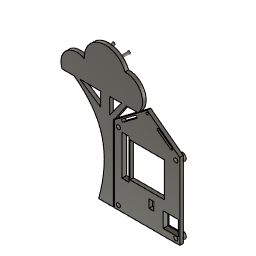
FaceCover v11 (Autodesk Fusion 360 design; units mm, degrees)
Autodesk Fusion 360 part; units mm, degrees
note: some values were not read from the file. Set by a fixed rule: which sketch regions a step uses.
sketch "House" plane through (0, 0, 0) normal (0, 1, 0) x (1, 0, 0)
  line L0 (27.95, 32.5) -> (-27.95, 32.5)
  line L1 (-27.95, 32.5) -> (-27.95, -32.5)
  line L2 (-27.95, -32.5) -> (27.95, -32.5)
  line L3 (27.95, -32.5) -> (27.95, 32.5)
  line L4 (27.95, 32.5) -> (-27.95, -32.5) construction
  line L5 (-27.95, 32.5) -> (27.95, -32.5) construction
  line L6 (14.8, 5.3) -> (-14.7, 5.3)
  line L7 (-14.7, 5.3) -> (-14.7, -24.2)
  line L8 (-14.7, -24.2) -> (14.8, -24.2)
  line L9 (14.8, -24.2) -> (14.8, 5.3)
  line L10 (14.8, 5.3) -> (-14.7, -24.2) construction
  line L11 (-14.7, 5.3) -> (14.8, -24.2) construction
  circle A0 centre (-24.45, 29) radius 1.75
  circle A1 centre (-24.45, -28.7) radius 1.75
  line L12 (-24.45, 29) -> (-24.45, -28.7) construction
  circle A2 centre (24.55, 29) radius 1.75
  line L13 (-24.45, 29) -> (24.55, 29) construction
  circle A3 centre (24.55, -28.7) radius 1.75
  line L14 (-24.45, -28.7) -> (24.55, -28.7) construction
  line L15 (24.55, -28.7) -> (24.55, 29) construction
  line L16 (-15.45, -24.5) -> (-19.45, -24.5)
  line L17 (-19.45, -24.5) -> (-19.45, 5.5)
  line L18 (-19.45, 5.5) -> (-15.45, 5.5)
  line L19 (-15.45, 5.5) -> (-15.45, -24.5)
  line L20 (15.7, 16) -> (24.7, 16)
  line L21 (24.7, 16) -> (24.7, 25)
  line L22 (24.7, 25) -> (15.7, 25)
  line L23 (15.7, 25) -> (15.7, 16)
  line L24 (1.65, 11.25) -> (5.65, 11.25)
  line L25 (5.65, 11.25) -> (5.65, 18.25)
  line L26 (5.65, 18.25) -> (1.65, 18.25)
  line L27 (1.65, 18.25) -> (1.65, 11.25)
  point P0 (0.05, -9.45)
  dimension "d1" = 55.9
  dimension "d2" = 65
  dimension "d3" = 29.5
  dimension "d4" = 29.5
  dimension "d5" = 27.2
  dimension "d7" = 3.5
  dimension "d8" = 3.5
  dimension "d10" = 57.7
  dimension "d12" = 49
  dimension "d13" = 3.5
  dimension "d14" = 4
  dimension "d15" = 30
  dimension "d16" = 8.5
  dimension "d17" = 27
  dimension "d18" = 9
  dimension "d19" = 9
  dimension "d20" = 7.5
  dimension "d21" = 3.25
  dimension "d22" = 4
  dimension "d23" = 7
  dimension "d24" = 14.25
  dimension "d25" = 22.3
  dimension "d92" = 28
  constraint horizontal L0
  constraint perpendicular L0 L1
  constraint parallel L0 L2
  constraint parallel L1 L3
  constraint coincident L4 origin
  constraint coincident L5 origin
  constraint horizontal L6
  constraint perpendicular L6 L7
  constraint parallel L6 L8
  constraint parallel L7 L9
  constraint coincident L10 P0
  constraint coincident L11 P0
  constraint coincident A0.centre L12.start
  constraint coincident A1.centre L12.end
  constraint vertical L12
  constraint coincident A2.centre L13.end
  constraint parallel L0 L13
  constraint coincident A3.centre L14.end
  constraint vertical L15
  constraint horizontal L16
  constraint vertical L17
  constraint horizontal L18
  constraint vertical L19
  constraint horizontal L20
  constraint vertical L21
  constraint horizontal L22
  constraint vertical L23
  constraint horizontal L24
  constraint vertical L25
  constraint horizontal L26
  constraint vertical L27
  constraint equal A1 A3
  constraint equal A0 A1
  constraint equal A0 A2
  measures "d1" distance of L1.end L2.end
  measures "d2" distance of L0.end L1.end
  measures "d3" distance of L7.end L8.end
  measures "d4" distance of L6.start L8.end
  measures "d5" distance of L0 L6
  measures "d7" distance of L0 A0.centre
  measures "d8" distance of L1 A0.centre
  measures "d10" distance of A0.centre A1.centre
  measures "d12" distance of A0.centre A2.centre
  measures "d13" diameter of A3
  measures "d14" distance of L16.start L16.end
  measures "d15" distance of L16.start L18.end
  measures "d16" distance of L1 L17
  measures "d17" distance of L0 L18
  measures "d18" distance of L20.start L20.end
  measures "d19" distance of L20.start L22.end
  measures "d20" distance of L0 L22
  measures "d21" distance of L3 L21
  measures "d22" distance of L24.start L24.end
  measures "d23" distance of L24.start L26.end
  measures "d24" distance of L0 L26
  measures "d25" distance of L3 L25
  measures "d92" distance of L1 P0
extrude "Extrude1" add sketch "House" along normal blind 3 makes body 1
sketch "Roof" plane through (0, 0, 0) normal (0, -1, 0) x (1, 0, 0)
  circle A0 centre (24.55, -29) radius 1.75
  line L0 (14.8, 24.2) -> (14.8, -5.3)
  line L1 (14.8, -5.3) -> (-14.7, -5.3)
  line L2 (-14.7, -5.3) -> (-14.7, 24.2)
  line L3 (-14.7, 24.2) -> (14.8, 24.2)
  circle A1 centre (-24.45, 28.7) radius 1.75
  circle A2 centre (-24.45, -29) radius 1.75
  circle A3 centre (24.55, 28.7) radius 1.75
  line L4 (-15.45, -5.5) -> (-19.45, -5.5)
  line L5 (-19.45, -5.5) -> (-19.45, 24.5)
  line L6 (-19.45, 24.5) -> (-15.45, 24.5)
  line L7 (-15.45, 24.5) -> (-15.45, -5.5)
  line L8 (15.7, -25) -> (15.7, -16)
  line L9 (15.7, -16) -> (24.7, -16)
  line L10 (24.7, -16) -> (24.7, -25)
  line L11 (24.7, -25) -> (15.7, -25)
  line L12 (1.65, -18.25) -> (1.65, -11.25)
  line L13 (1.65, -11.25) -> (5.65, -11.25)
  line L14 (5.65, -11.25) -> (5.65, -18.25)
  line L15 (5.65, -18.25) -> (1.65, -18.25)
  line L16 (27.95, -32.5) -> (27.95, 32.5)
  line L17 (27.95, 32.5) -> (-27.95, 32.5)
  line L18 (-27.95, 32.5) -> (-27.95, -32.5)
  line L19 (-27.95, -32.5) -> (27.95, -32.5)
  line L20 (-27.95, 32.5) -> (0, 53.5)
  line L21 (0, 53.5) -> (27.95, 32.5)
  line L22 (0, 0) -> (0, 2.2581) construction
  line L23 (0, 2.2581) -> (0, 69.3742) construction
  dimension "d28" = 21
  constraint coincident L17.end L18.start
  constraint coincident L16.end L17.start
  constraint coincident L22.start origin
  constraint perpendicular L1 L22
  constraint parallel L0 L23
  constraint coincident L20.end L23
  measures "d28" distance of L17 L20.end
extrude "Extrude2" add sketch "Roof" against normal blind 3 contours L17 L20 L21 bodies 1
sketch "Chimney" plane through (0, 0, 0) normal (0, -1, 0) x (1, 0, 0)
  circle A0 centre (24.55, -29) radius 1.75
  line L0 (14.8, 24.2) -> (14.8, -5.3)
  line L1 (14.8, -5.3) -> (-14.7, -5.3)
  line L2 (-14.7, -5.3) -> (-14.7, 24.2)
  line L3 (-14.7, 24.2) -> (14.8, 24.2)
  circle A1 centre (-24.45, 28.7) radius 1.75
  circle A2 centre (-24.45, -29) radius 1.75
  circle A3 centre (24.55, 28.7) radius 1.75
  line L4 (-15.45, -5.5) -> (-19.45, -5.5)
  line L5 (-19.45, -5.5) -> (-19.45, 24.5)
  line L6 (-19.45, 24.5) -> (-15.45, 24.5)
  line L7 (-15.45, 24.5) -> (-15.45, -5.5)
  line L8 (15.7, -25) -> (15.7, -16)
  line L9 (15.7, -16) -> (24.7, -16)
  line L10 (24.7, -16) -> (24.7, -25)
  line L11 (24.7, -25) -> (15.7, -25)
  line L12 (1.65, -18.25) -> (1.65, -11.25)
  line L13 (1.65, -11.25) -> (5.65, -11.25)
  line L14 (5.65, -11.25) -> (5.65, -18.25)
  line L15 (5.65, -18.25) -> (1.65, -18.25)
  line L16 (27.95, -32.5) -> (27.95, 32.5)
  line L17 (27.95, 32.5) -> (0, 53.5)
  line L18 (0, 53.5) -> (-27.95, 32.5)
  line L19 (-27.95, 32.5) -> (-27.95, -32.5)
  line L20 (-27.95, -32.5) -> (27.95, -32.5)
  line L21 (-3, 43.5) -> (-21, 43.5)
  line L22 (-21, 43.5) -> (-21, 69.5)
  line L23 (-21, 69.5) -> (-3, 69.5)
  line L24 (-3, 69.5) -> (-3, 43.5)
  line L25 (-3, 43.5) -> (-21, 69.5) construction
  line L26 (-21, 43.5) -> (-3, 69.5) construction
  point P0 (-12, 56.5)
  dimension "d31" = 18
  dimension "d32" = 26
  dimension "d33" = 76
  dimension "d34" = 3
  constraint horizontal L21
  constraint perpendicular L21 L22
  constraint parallel L21 L23
  constraint parallel L22 L24
  constraint coincident L25 P0
  constraint coincident L26 P0
  measures "d31" distance of L22.end L23.end
  measures "d32" distance of L21.end L22.end
  measures "d33" distance of L20 L21
  measures "d34" distance of origin L24
extrude "Extrude3" add sketch "Chimney" against normal blind 3 contours L18 L21 L22 L23 L24 bodies 1
sketch "Chimney2" plane through (0, 0, 0) normal (0, -1, 0) x (1, 0, 0)
  circle A0 centre (24.55, -29) radius 1.75
  line L0 (14.8, 24.2) -> (14.8, -5.3)
  line L1 (14.8, -5.3) -> (-14.7, -5.3)
  line L2 (-14.7, -5.3) -> (-14.7, 24.2)
  line L3 (-14.7, 24.2) -> (14.8, 24.2)
  circle A1 centre (-24.45, 28.7) radius 1.75
  circle A2 centre (-24.45, -29) radius 1.75
  circle A3 centre (24.55, 28.7) radius 1.75
  line L4 (-15.45, -5.5) -> (-19.45, -5.5)
  line L5 (-19.45, -5.5) -> (-19.45, 24.5)
  line L6 (-19.45, 24.5) -> (-15.45, 24.5)
  line L7 (-15.45, 24.5) -> (-15.45, -5.5)
  line L8 (15.7, -25) -> (15.7, -16)
  line L9 (15.7, -16) -> (24.7, -16)
  line L10 (24.7, -16) -> (24.7, -25)
  line L11 (24.7, -25) -> (15.7, -25)
  line L12 (1.65, -18.25) -> (1.65, -11.25)
  line L13 (1.65, -11.25) -> (5.65, -11.25)
  line L14 (5.65, -11.25) -> (5.65, -18.25)
  line L15 (5.65, -18.25) -> (1.65, -18.25)
  line L16 (27.95, -32.5) -> (27.95, 32.5)
  line L17 (27.95, 32.5) -> (0, 53.5)
  line L18 (0, 53.5) -> (-3, 51.246)
  line L19 (-3, 51.246) -> (-3, 69.5)
  line L20 (-3, 69.5) -> (-21, 69.5)
  line L21 (-21, 69.5) -> (-21, 43.5)
  line L22 (-21, 43.5) -> (-13.3095, 43.5)
  line L23 (-13.3095, 43.5) -> (-27.95, 32.5)
  line L24 (-27.95, 32.5) -> (-27.95, -32.5)
  line L25 (-27.95, -32.5) -> (27.95, -32.5)
  line L26 (-21, 43.5) -> (-21, 37.7218)
  constraint coincident L21.end L22.start
  constraint coincident L23 L26.end
  constraint perpendicular L22 L26
extrude "Extrude4" add sketch "Chimney2" against normal up to surface (3 mm away) contours L22 L23 L26 bodies 1
sketch "Pegs1" plane through (0, 3, 0) normal (0, 1, 0) x (-1, 0, 0)
  circle A0 centre (-24.55, -29) radius 1.75
  line L0 (-14.8, -5.3) -> (-14.8, 24.2)
  line L1 (-14.8, 24.2) -> (14.7, 24.2)
  line L2 (14.7, 24.2) -> (14.7, -5.3)
  line L3 (14.7, -5.3) -> (-14.8, -5.3)
  circle A1 centre (24.45, 28.7) radius 1.75
  circle A2 centre (24.45, -29) radius 1.75
  circle A3 centre (-24.55, 28.7) radius 1.75
  line L4 (19.45, -5.5) -> (15.45, -5.5)
  line L5 (15.45, -5.5) -> (15.45, 24.5)
  line L6 (15.45, 24.5) -> (19.45, 24.5)
  line L7 (19.45, 24.5) -> (19.45, -5.5)
  line L8 (-15.7, -16) -> (-15.7, -25)
  line L9 (-15.7, -25) -> (-24.7, -25)
  line L10 (-24.7, -25) -> (-24.7, -16)
  line L11 (-24.7, -16) -> (-15.7, -16)
  line L12 (-1.65, -11.25) -> (-1.65, -18.25)
  line L13 (-1.65, -18.25) -> (-5.65, -18.25)
  line L14 (-5.65, -18.25) -> (-5.65, -11.25)
  line L15 (-5.65, -11.25) -> (-1.65, -11.25)
  line L16 (-27.95, 32.5) -> (-27.95, -32.5)
  line L17 (-27.95, -32.5) -> (27.95, -32.5)
  line L18 (27.95, -32.5) -> (27.95, 32.5)
  line L19 (27.95, 32.5) -> (21, 37.7218)
  line L20 (21, 37.7218) -> (21, 69.5)
  line L21 (21, 69.5) -> (3, 69.5)
  line L22 (3, 69.5) -> (3, 51.246)
  line L23 (3, 51.246) -> (0, 53.5)
  line L24 (0, 53.5) -> (-27.95, 32.5)
  circle A4 centre (5.5, 67) radius 1.15
  circle A5 centre (18.5, 67) radius 1.15
  circle A6 centre (18.5, 46.5) radius 1.15
  line L25 (5.5, 67) -> (18.5, 67) construction
  line L26 (18.5, 67) -> (18.5, 46.5) construction
  line L27 (18.5, 46.5) -> (5.5, 46.5) construction
  line L28 (5.5, 46.5) -> (5.5, 67) construction
  line L29 (12, 69.5) -> (12, 42.8534) construction
  dimension "d39" = 2.3
  dimension "d40" = 13
  dimension "d41" = 20.5
  dimension "d42" = 2.5
  constraint equal A4 A5
  constraint equal A5 A6
  constraint coincident A4.centre L25.start
  constraint coincident A5.centre L25.end
  constraint coincident A6.centre L26.end
  constraint vertical L26
  constraint horizontal L25
  constraint horizontal L27
  constraint midpoint L21 L29.start
  constraint symmetric A4 A5 L29
  constraint vertical L28
  measures "d39" diameter of A4
  measures "d40" distance of A4.centre A5.centre
  measures "d41" distance of A5.centre A6.centre
  measures "d42" distance of L21 L25
extrude "Extrude5" add sketch "Pegs1" along normal blind 10 contours A4 | A5 | A6 bodies 1
sketch "StandOffs" plane through (0, 3, 0) normal (0, 1, 0) x (-1, 0, 0)
  line L0 (-1.65, -11.25) -> (-1.65, -18.25)
  line L1 (-1.65, -18.25) -> (-5.65, -18.25)
  line L2 (-5.65, -18.25) -> (-5.65, -11.25)
  line L3 (-5.65, -11.25) -> (-1.65, -11.25)
  line L4 (-14.8, -5.3) -> (-14.8, 24.2)
  line L5 (-14.8, 24.2) -> (14.7, 24.2)
  line L6 (14.7, 24.2) -> (14.7, -5.3)
  line L7 (14.7, -5.3) -> (-14.8, -5.3)
  line L8 (-15.7, -16) -> (-15.7, -25)
  line L9 (-15.7, -25) -> (-24.7, -25)
  line L10 (-24.7, -25) -> (-24.7, -16)
  line L11 (-24.7, -16) -> (-15.7, -16)
  line L12 (19.45, -5.5) -> (15.45, -5.5)
  line L13 (15.45, -5.5) -> (15.45, 24.5)
  line L14 (15.45, 24.5) -> (19.45, 24.5)
  line L15 (19.45, 24.5) -> (19.45, -5.5)
  circle A0 centre (-24.55, 28.7) radius 1.75
  circle A1 centre (24.45, -29) radius 1.75
  circle A2 centre (24.45, 28.7) radius 1.75
  circle A3 centre (-24.55, -29) radius 1.75
  line L16 (-27.95, 32.5) -> (-27.95, -32.5)
  line L17 (-27.95, -32.5) -> (27.95, -32.5)
  line L18 (27.95, -32.5) -> (27.95, 32.5)
  line L19 (27.95, 32.5) -> (21, 37.7218)
  line L20 (21, 37.7218) -> (21, 69.5)
  line L21 (21, 69.5) -> (3, 69.5)
  line L22 (3, 69.5) -> (3, 51.246)
  line L23 (3, 51.246) -> (0, 53.5)
  line L24 (0, 53.5) -> (-27.95, 32.5)
  circle A4 centre (-24.55, 28.7) radius 3.25
  circle A5 centre (24.45, 28.7) radius 3.25
  circle A6 centre (-24.55, -29) radius 3.25
  circle A7 centre (24.45, -29) radius 3.25
  circle A8 centre (18.5, 46.5) radius 1.15
  circle A9 centre (18.5, 67) radius 1.15
  circle A10 centre (5.5, 67) radius 1.15
  dimension "d45" = 1.5
  dimension "d46" = 1.5
  dimension "d47" = 1.5
  dimension "d48" = 1.5
extrude "Extrude6" add sketch "StandOffs" along normal blind 2.6 contours A4 | A5 | A6 | A7 bodies 1
sketch "DotstarSlot" plane through (0, 0, 0) normal (0, -1, 0) x (1, 0, 0)
  line L0 (1.65, -18.25) -> (1.65, -11.25)
  line L1 (1.65, -11.25) -> (5.65, -11.25)
  line L2 (5.65, -11.25) -> (5.65, -18.25)
  line L3 (5.65, -18.25) -> (1.65, -18.25)
  line L4 (14.8, 24.2) -> (14.8, -5.3)
  line L5 (14.8, -5.3) -> (-14.7, -5.3)
  line L6 (-14.7, -5.3) -> (-14.7, 24.2)
  line L7 (-14.7, 24.2) -> (14.8, 24.2)
  line L8 (15.7, -25) -> (15.7, -16)
  line L9 (15.7, -16) -> (24.7, -16)
  line L10 (24.7, -16) -> (24.7, -25)
  line L11 (24.7, -25) -> (15.7, -25)
  line L12 (-15.45, -5.5) -> (-19.45, -5.5)
  line L13 (-19.45, -5.5) -> (-19.45, 24.5)
  line L14 (-19.45, 24.5) -> (-15.45, 24.5)
  line L15 (-15.45, 24.5) -> (-15.45, -5.5)
  circle A0 centre (24.55, 28.7) radius 1.75
  circle A1 centre (-24.45, -29) radius 1.75
  circle A2 centre (-24.45, 28.7) radius 1.75
  circle A3 centre (24.55, -29) radius 1.75
  line L16 (27.95, -32.5) -> (27.95, 32.5)
  line L17 (27.95, 32.5) -> (0, 53.5)
  line L18 (0, 53.5) -> (-3, 51.246)
  line L19 (-3, 51.246) -> (-3, 69.5)
  line L20 (-3, 69.5) -> (-21, 69.5)
  line L21 (-21, 69.5) -> (-21, 37.7218)
  line L22 (-21, 37.7218) -> (-27.95, 32.5)
  line L23 (-27.95, 32.5) -> (-27.95, -32.5)
  line L24 (-27.95, -32.5) -> (27.95, -32.5)
  line L25 (-20.1859, 34.5811) -> (-8.9931, 42.9907)
  arc A4 (-8.9931, 42.9907) -> (-10.1945, 44.5896) centre (-9.5938, 43.7902) ccw
  line L26 (-10.1945, 44.5896) -> (-21.3873, 36.18)
  arc A5 (-21.3873, 36.18) -> (-20.1859, 34.5811) centre (-20.7866, 35.3805) ccw
  line L27 (-20.7866, 35.3805) -> (0, 50.9984) construction
  line L28 (0, 0) -> (0, 53.5) construction
  dimension "d51" = 1
  dimension "d52" = 2
  dimension "d53" = 26
  dimension "d57" = 14
  constraint tangent L25 A4
  constraint tangent A4 L26
  constraint parallel L25 L26
  constraint tangent L26 A5
  constraint tangent L25 A5
  constraint parallel L22 L27
  constraint coincident L28.start origin
  constraint coincident L17.end L18.start
  constraint coincident L27.end L28
  constraint coincident L27 A4.centre
  measures "d51" radius of A5
  measures "d52" distance of L22 L27
  measures "d53" distance of A5.centre L27.end
  measures "d57" distance of A5.centre A4.centre
extrude "Extrude7" cut sketch "DotstarSlot" against normal through all contours L25 A4 L26 A5 bodies 1
mirror "Mirror1" about plane through (0, 0, 0) normal (1, 0, 0) of "Extrude7"
sketch "DotstarHole" plane through (0, 0, 0) normal (0, -1, 0) x (1, 0, 0)
  line L0 (20.1859, 34.5811) -> (8.9931, 42.9907)
  arc A0 (10.1945, 44.5896) -> (8.9931, 42.9907) centre (9.5938, 43.7902) ccw
  line L1 (10.1945, 44.5896) -> (21.3873, 36.18)
  arc A1 (20.1859, 34.5811) -> (21.3873, 36.18) centre (20.7866, 35.3805) ccw
  line L2 (-21.3873, 36.18) -> (-10.1945, 44.5896)
  arc A2 (-8.9931, 42.9907) -> (-10.1945, 44.5896) centre (-9.5938, 43.7902) ccw
  line L3 (-8.9931, 42.9907) -> (-20.1859, 34.5811)
  arc A3 (-21.3873, 36.18) -> (-20.1859, 34.5811) centre (-20.7866, 35.3805) ccw
  line L4 (1.65, -18.25) -> (1.65, -11.25)
  line L5 (1.65, -11.25) -> (5.65, -11.25)
  line L6 (5.65, -11.25) -> (5.65, -18.25)
  line L7 (5.65, -18.25) -> (1.65, -18.25)
  line L8 (14.8, 24.2) -> (14.8, -5.3)
  line L9 (14.8, -5.3) -> (-14.7, -5.3)
  line L10 (-14.7, -5.3) -> (-14.7, 24.2)
  line L11 (-14.7, 24.2) -> (14.8, 24.2)
  line L12 (15.7, -25) -> (15.7, -16)
  line L13 (15.7, -16) -> (24.7, -16)
  line L14 (24.7, -16) -> (24.7, -25)
  line L15 (24.7, -25) -> (15.7, -25)
  line L16 (-15.45, -5.5) -> (-19.45, -5.5)
  line L17 (-19.45, -5.5) -> (-19.45, 24.5)
  line L18 (-19.45, 24.5) -> (-15.45, 24.5)
  line L19 (-15.45, 24.5) -> (-15.45, -5.5)
  circle A4 centre (24.55, 28.7) radius 1.75
  circle A5 centre (-24.45, -29) radius 1.75
  circle A6 centre (-24.45, 28.7) radius 1.75
  circle A7 centre (24.55, -29) radius 1.75
  line L20 (27.95, -32.5) -> (27.95, 32.5)
  line L21 (27.95, 32.5) -> (0, 53.5)
  line L22 (0, 53.5) -> (-3, 51.246)
  line L23 (-3, 51.246) -> (-3, 69.5)
  line L24 (-3, 69.5) -> (-21, 69.5)
  line L25 (-21, 69.5) -> (-21, 37.7218)
  line L26 (-21, 37.7218) -> (-27.95, 32.5)
  line L27 (-27.95, 32.5) -> (-27.95, -32.5)
  line L28 (-27.95, -32.5) -> (27.95, -32.5)
  line L29 (0, 0) -> (0, 53.5) construction
  circle A8 centre (0, 51) radius 1
  dimension "d58" = 2
  dimension "d59" = 2.5
  constraint coincident L29.start origin
  constraint coincident L21.end L22.start
  constraint coincident L29 A8.centre
  measures "d58" diameter of A8
  measures "d59" distance of L21.end A8.centre
extrude "Extrude8" cut sketch "DotstarHole" against normal through all contours A8 bodies 1
chamfer "Chamfer1" distance 2 angle 45 4 edges at (20.2, 0, -16) (24.7, 0, -20.5) (20.2, 0, -25) (15.7, 0, -20.5) on bodies 1
chamfer "Chamfer2" distance 2 angle 45 3 edges at (-17.45, 0, 24.5) (-19.45, 0, 9.5) (-17.45, 0, -5.5) on bodies 1
sketch "ButtonRelief" plane through (0, 3, 0) normal (0, 1, 0) x (-1, 0, 0)
  circle A0 centre (0, 51) radius 1
  line L0 (-8.9931, 42.9907) -> (-20.1859, 34.5811)
  arc A1 (-21.3873, 36.18) -> (-20.1859, 34.5811) centre (-20.7866, 35.3805) ccw
  line L1 (-21.3873, 36.18) -> (-10.1945, 44.5896)
  arc A2 (-8.9931, 42.9907) -> (-10.1945, 44.5896) centre (-9.5938, 43.7902) ccw
  line L2 (10.1945, 44.5896) -> (21.3873, 36.18)
  arc A3 (20.1859, 34.5811) -> (21.3873, 36.18) centre (20.7866, 35.3805) ccw
  line L3 (20.1859, 34.5811) -> (8.9931, 42.9907)
  arc A4 (10.1945, 44.5896) -> (8.9931, 42.9907) centre (9.5938, 43.7902) ccw
  circle A5 centre (24.45, -29) radius 3.25
  circle A6 centre (-24.55, 28.7) radius 3.25
  circle A7 centre (-24.55, -29) radius 3.25
  circle A8 centre (24.45, 28.7) radius 3.25
  line L4 (-14.8, -5.3) -> (-14.8, 24.2)
  line L5 (-14.8, 24.2) -> (14.7, 24.2)
  line L6 (14.7, 24.2) -> (14.7, -5.3)
  line L7 (14.7, -5.3) -> (-14.8, -5.3)
  line L8 (-1.65, -11.25) -> (-1.65, -18.25)
  line L9 (-1.65, -18.25) -> (-5.65, -18.25)
  line L10 (-5.65, -18.25) -> (-5.65, -11.25)
  line L11 (-5.65, -11.25) -> (-1.65, -11.25)
  line L12 (-15.7, -16) -> (-15.7, -25)
  line L13 (-15.7, -25) -> (-24.7, -25)
  line L14 (-24.7, -25) -> (-24.7, -16)
  line L15 (-24.7, -16) -> (-15.7, -16)
  line L16 (19.45, -5.5) -> (15.45, -5.5)
  line L17 (15.45, -5.5) -> (15.45, 24.5)
  line L18 (15.45, 24.5) -> (19.45, 24.5)
  line L19 (19.45, 24.5) -> (19.45, -5.5)
  line L20 (-27.95, 32.5) -> (-27.95, -32.5)
  line L21 (-27.95, -32.5) -> (27.95, -32.5)
  line L22 (27.95, -32.5) -> (27.95, 32.5)
  line L23 (27.95, 32.5) -> (21, 37.7218)
  line L24 (21, 37.7218) -> (21, 69.5)
  line L25 (21, 69.5) -> (3, 69.5)
  line L26 (3, 69.5) -> (3, 51.246)
  line L27 (3, 51.246) -> (0, 53.5)
  line L28 (0, 53.5) -> (-27.95, 32.5)
  line L29 (15.45, 24.5) -> (15.45, 26)
  line L30 (15.45, 26) -> (20.95, 26)
  line L31 (20.95, 26) -> (20.95, -7)
  line L32 (20.95, -7) -> (15.45, -7)
  line L33 (15.45, -7) -> (15.45, -5.5)
  circle A9 centre (18.5, 46.5) radius 1.15
  circle A10 centre (18.5, 67) radius 1.15
  circle A11 centre (5.5, 67) radius 1.15
  dimension "d64" = 33
  dimension "d65" = 5.5
  constraint coincident L17.end L18.start
  constraint perpendicular L18 L29
  constraint perpendicular L29 L30
  constraint perpendicular L30 L31
  constraint perpendicular L31 L32
  constraint coincident L16.end L17.start
  constraint perpendicular L16 L33
  constraint equal L29 L33
  measures "d64" distance of L30.end L31.end
  measures "d65" distance of L31.end L32.end
extrude "Extrude9" cut sketch "ButtonRelief" against normal blind 1 contours L16 L18 L19 L29 L30 L31 L32 L33 bodies 1
sketch "CutChimney" plane through (0, 0, 0) normal (0, -1, 0) x (1, 0, 0)
  line L0 (26.7, -14) -> (26.7, -27)
  line L1 (26.7, -27) -> (13.7, -27)
  line L2 (13.7, -27) -> (13.7, -14)
  line L3 (13.7, -14) -> (26.7, -14)
  circle A0 centre (0, 51) radius 1
  line L4 (20.1859, 34.5811) -> (8.9931, 42.9907)
  arc A1 (10.1945, 44.5896) -> (8.9931, 42.9907) centre (9.5938, 43.7902) ccw
  line L5 (10.1945, 44.5896) -> (21.3873, 36.18)
  arc A2 (20.1859, 34.5811) -> (21.3873, 36.18) centre (20.7866, 35.3805) ccw
  line L6 (-21.3873, 36.18) -> (-10.1945, 44.5896)
  arc A3 (-8.9931, 42.9907) -> (-10.1945, 44.5896) centre (-9.5938, 43.7902) ccw
  line L7 (-8.9931, 42.9907) -> (-20.1859, 34.5811)
  arc A4 (-21.3873, 36.18) -> (-20.1859, 34.5811) centre (-20.7866, 35.3805) ccw
  circle A5 centre (24.55, 28.7) radius 1.75
  circle A6 centre (24.55, -29) radius 1.75
  circle A7 centre (-24.45, 28.7) radius 1.75
  line L8 (14.8, 24.2) -> (14.8, -5.3)
  line L9 (14.8, -5.3) -> (-14.7, -5.3)
  line L10 (-14.7, -5.3) -> (-14.7, 24.2)
  line L11 (-14.7, 24.2) -> (14.8, 24.2)
  line L12 (1.65, -18.25) -> (1.65, -11.25)
  line L13 (1.65, -11.25) -> (5.65, -11.25)
  line L14 (5.65, -11.25) -> (5.65, -18.25)
  line L15 (5.65, -18.25) -> (1.65, -18.25)
  line L16 (-15.45, 26.5) -> (-15.45, -7.5)
  line L17 (-15.45, -7.5) -> (-21.45, -7.5)
  line L18 (-21.45, -7.5) -> (-21.45, 26.5)
  line L19 (-21.45, 26.5) -> (-15.45, 26.5)
  circle A8 centre (-24.45, -29) radius 1.75
  line L20 (27.95, -32.5) -> (27.95, 32.5)
  line L21 (27.95, 32.5) -> (0, 53.5)
  line L22 (0, 53.5) -> (-3, 51.246)
  line L23 (-3, 51.246) -> (-3, 69.5)
  line L24 (-3, 69.5) -> (-21, 69.5)
  line L25 (-21, 69.5) -> (-21, 37.7218)
  line L26 (-21, 37.7218) -> (-27.95, 32.5)
  line L27 (-27.95, 32.5) -> (-27.95, -32.5)
  line L28 (-27.95, -32.5) -> (27.95, -32.5)
  line L29 (-21, 37.7218) -> (-3, 51.246)
  constraint coincident L25.end L26.start
  constraint coincident L22.end L23.start
extrude "CutChimney (1)" cut sketch "CutChimney" against normal through all contours L23 L24 L25 L29 bodies 1
sketch "Tree" plane through (0, 0, 0) normal (0, -1, 0) x (1, 0, 0)
  line L0 (0, 53.5) -> (-27.95, 32.5)
  line L1 (-27.95, 32.5) -> (-27.95, -32.5)
  line L2 (-27.95, -32.5) -> (27.95, -32.5)
  line L3 (27.95, -32.5) -> (27.95, 32.5)
  line L4 (27.95, 32.5) -> (0, 53.5)
  line L5 (26.7, -14) -> (26.7, -27)
  line L6 (26.7, -27) -> (13.7, -27)
  line L7 (13.7, -27) -> (13.7, -14)
  line L8 (13.7, -14) -> (26.7, -14)
  circle A0 centre (0, 51) radius 1
  line L9 (20.1859, 34.5811) -> (8.9931, 42.9907)
  arc A1 (10.1945, 44.5896) -> (8.9931, 42.9907) centre (9.5938, 43.7902) ccw
  line L10 (10.1945, 44.5896) -> (21.3873, 36.18)
  arc A2 (20.1859, 34.5811) -> (21.3873, 36.18) centre (20.7866, 35.3805) ccw
  line L11 (-21.3873, 36.18) -> (-10.1945, 44.5896)
  arc A3 (-8.9931, 42.9907) -> (-10.1945, 44.5896) centre (-9.5938, 43.7902) ccw
  line L12 (-8.9931, 42.9907) -> (-20.1859, 34.5811)
  arc A4 (-21.3873, 36.18) -> (-20.1859, 34.5811) centre (-20.7866, 35.3805) ccw
  circle A5 centre (24.55, 28.7) radius 1.75
  circle A6 centre (24.55, -29) radius 1.75
  circle A7 centre (-24.45, 28.7) radius 1.75
  line L13 (14.8, 24.2) -> (14.8, -5.3)
  line L14 (14.8, -5.3) -> (-14.7, -5.3)
  line L15 (-14.7, -5.3) -> (-14.7, 24.2)
  line L16 (-14.7, 24.2) -> (14.8, 24.2)
  line L17 (1.65, -18.25) -> (1.65, -11.25)
  line L18 (1.65, -11.25) -> (5.65, -11.25)
  line L19 (5.65, -11.25) -> (5.65, -18.25)
  line L20 (5.65, -18.25) -> (1.65, -18.25)
  line L21 (-15.45, 26.5) -> (-15.45, -7.5)
  line L22 (-15.45, -7.5) -> (-21.45, -7.5)
  line L23 (-21.45, -7.5) -> (-21.45, 26.5)
  line L24 (-21.45, 26.5) -> (-15.45, 26.5)
  circle A8 centre (-24.45, -29) radius 1.75
  line L25 (-7.6474, 47.7542) -> (-72.5425, 47.7542)
  circle A9 centre (-35.5908, 65.8795) radius 18.0148
  arc A10 (-47.2723, 47.7542) -> (-72.5425, 47.7542) centre (-59.9074, 52.8008) ccw
  arc A11 (-7.6474, 47.7542) -> (-29.2007, 47.7542) centre (-18.424, 57.7206) ccw
  spline S0 degree 5 poles (-62.2442, 47.7542) (-60.7892, 46.6894) (-57.9722, 44.5111) (-54.0263, 41.098) (-49.3332, 36.2509) (-44.4754, 29.6661) (-40.7068, 22.5133) (-38.1015, 14.7539) (-36.6724, 6.3812) (-36.3462, -2.5667) (-37.0276, -12.0399) (-38.3069, -20.0014) (-39.6523, -26.1738) (-40.7178, -30.3766) (-41.2928, -32.5) knots 0 0 0 0 0 0 0.1 0.2 0.3 0.4 0.5 0.6 0.7 0.8 0.9 1 1 1 1 1 1
  line L26 (-41.2928, -32.5) -> (-27.95, -32.5)
  line L27 (-57.2922, 47.7542) -> (-39.6559, 36.0437)
  line L28 (-39.6559, 36.0437) -> (-39.6559, 47.7542)
  line L29 (-31.8322, 47.7542) -> (-31.8322, 34.0546)
  line L30 (-31.8322, 34.0546) -> (-21.887, 47.7542)
  line L31 (-17.5567, 47.7542) -> (-27.95, 32.5)
  line L32 (-3, 50.3533) -> (-27.95, 32.5)
  line L33 (-27.95, -32.5) -> (-27.95, 32.5)
  point P0 (-39.0798, 17.0814)
  constraint coincident L0 L25.start
  constraint horizontal L25
  constraint coincident L25 A10.start
  constraint coincident L25 A11.end
  constraint coincident L25 S0.start
  constraint coincident L1.end L2.start
  constraint perpendicular L1 L26
  constraint coincident L25 L27.start
  constraint coincident L25 L28.end
  constraint perpendicular L25 L28
  constraint coincident L25 L29.start
  constraint perpendicular L25 L29
  constraint coincident L25 L30.end
  constraint coincident L25 L31.start
  constraint coincident L31 L0.end
  constraint coincident L0.end L1.start
extrude "Ext_Tree" add sketch "Tree" against normal up to surface (3 mm away) separate body contours L25 A9 A11 | L1 L25 S0 L26 L27 L28 L29 L30 L31 L33 | A9 A10 A11 | A9 A11 | A9 A10 | L25 A9 A10 | L25 A9 A10 A11 makes body 2
sketch "OutlineHouse" plane through (0, 0, 0) normal (0, -1, 0) x (1, 0, 0)
  line L0 (-21.887, 47.7542) -> (-31.8322, 34.0546)
  line L1 (-31.8322, 34.0546) -> (-31.8322, 47.7542)
  line L2 (-31.8322, 47.7542) -> (-21.887, 47.7542)
  line L3 (-39.6559, 47.7542) -> (-39.6559, 36.0437)
  line L4 (-39.6559, 36.0437) -> (-57.2922, 47.7542)
  line L5 (-57.2922, 47.7542) -> (-39.6559, 47.7542)
  spline S0 degree 5 poles (-62.2442, 47.7542) (-60.7892, 46.6894) (-57.9722, 44.5111) (-54.0263, 41.098) (-49.3332, 36.2509) (-44.4754, 29.6661) (-40.7068, 22.5133) (-38.1015, 14.7539) (-36.6724, 6.3812) (-36.3462, -2.5667) (-37.0276, -12.0399) (-38.3069, -20.0014) (-39.6523, -26.1738) (-40.7178, -30.3766) (-41.2928, -32.5) knots 0 0 0 0 0 0 0.1 0.2 0.3 0.4 0.5 0.6 0.7 0.8 0.9 1 1 1 1 1 1
  line L6 (-41.2928, -32.5) -> (-27.95, -32.5)
  line L7 (-27.95, -32.5) -> (-27.95, 32.5)
  arc A0 (-7.6474, 47.7542) -> (-18.7954, 72.3947) centre (-18.424, 57.7206) ccw
  arc A1 (-18.7954, 72.3947) -> (-53.5758, 64.8433) centre (-35.5908, 65.8795) ccw
  arc A2 (-53.5758, 64.8433) -> (-72.5425, 47.7542) centre (-59.9074, 52.8008) ccw
  line L8 (-72.5425, 47.7542) -> (-62.2442, 47.7542)
  line L9 (-6.6322, 47.7542) -> (-27.95, 32.5)
  line L10 (-27.95, 32.5) -> (-27.95, -32.5)
  line L11 (-28.75, -32.5) -> (-28.75, 32.5)
  line L12 (-28.75, 32.5) -> (-6.6322, 47.7542)
  line L13 (-27.95, 32.5) -> (-17.5567, 47.7542)
  line L14 (-17.5567, 47.7542) -> (-7.6474, 47.7542)
  dimension "d78" = 0.8
  constraint coincident L7.end L9.end
  constraint coincident L6.end L7.start
  constraint coincident L6 L11.start
  constraint perpendicular L6 L11
  constraint equal L10 L11
  measures "d78" distance of L10 L11
extrude "Extrude13" cut sketch "OutlineHouse" against normal blind 0.8 contours L6 L7 L10 L11 L12 L13 bodies 2
chamfer "Chamfer4" distance 0.8 angle 45 1 edges at (-28.75, 0.8, 0) on bodies 2
sketch "Pegs2" plane through (0, 3, 0) normal (0, 1, 0) x (-1, 0, 0)
  line L0 (27.95, -32.5) -> (41.2928, -32.5)
  spline S0 degree 3 poles (62.2442, 47.7542) (56.8809, 43.8292) (49.9789, 37.8698) (40.9726, 23.5016) (38.6175, 17.0977) (36.3672, 3.4599) (36.388, -3.3723) (37.7522, -17.5261) (39.3157, -25.1981) (41.2928, -32.5) knots 0 0 0 0 1.993824 1.993824 3.434395 3.434395 4.784945 4.784945 6.320225 6.320225 6.320225 6.320225
  line L1 (62.2442, 47.7542) -> (72.5425, 47.7542)
  arc A0 (72.5425, 47.7542) -> (53.5758, 64.8433) centre (59.9074, 52.8008) ccw
  arc A1 (53.5758, 64.8433) -> (18.7954, 72.3947) centre (35.5908, 65.8795) ccw
  arc A2 (18.7954, 72.3947) -> (7.6474, 47.7542) centre (18.424, 57.7206) ccw
  line L2 (27.95, 32.5) -> (27.95, -32.5)
  line L3 (39.6559, 36.0437) -> (39.6559, 47.7542)
  line L4 (39.6559, 47.7542) -> (57.2922, 47.7542)
  line L5 (57.2922, 47.7542) -> (39.6559, 36.0437)
  line L6 (31.8322, 34.0546) -> (21.887, 47.7542)
  line L7 (21.887, 47.7542) -> (31.8322, 47.7542)
  line L8 (31.8322, 47.7542) -> (31.8322, 34.0546)
  line L9 (28.5, 75.5) -> (41.5, 75.5) construction
  line L10 (41.5, 75.5) -> (41.5, 55) construction
  line L11 (41.5, 55) -> (28.5, 55) construction
  line L12 (28.5, 55) -> (28.5, 75.5) construction
  circle A3 centre (28.5, 75.5) radius 1.15
  circle A4 centre (41.5, 75.5) radius 1.15
  circle A5 centre (41.5, 55) radius 1.15
  circle A6 centre (28.5, 55) radius 1.15
  line L13 (7.6474, 47.7542) -> (17.5567, 47.7542)
  line L14 (17.5567, 47.7542) -> (27.95, 32.5)
  dimension "d84" = 13
  dimension "d85" = 20.5
  dimension "d86" = 28.5
  dimension "d87" = 55
  dimension "d88" = 2.3
  constraint horizontal L9
  constraint perpendicular L9 L10
  constraint perpendicular L10 L11
  constraint perpendicular L9 L12
  constraint coincident L9.start L12.end
  constraint coincident L9.end L10.start
  constraint coincident L10.end L11.start
  constraint coincident L11.end L12.start
  constraint equal A3 A4
  constraint equal A4 A5
  constraint equal A5 A6
  measures "d84" distance of L9.start L9.end
  measures "d85" distance of L9.end L10.end
  measures "d86" distance of origin L12
  measures "d87" distance of origin L11
  measures "d88" diameter of A3
extrude "Extrude14" add sketch "Pegs2" along normal blind 10 contours A3 | A4 | A5 | A6 bodies 2
equation "d5 = Window_V"
equation "d92 = Window_H"
equation "Window_H = 28 mm" comment "Move Window Horizontally"
equation "Window_V = 27.2 mm" comment "Move Window Vertically"
